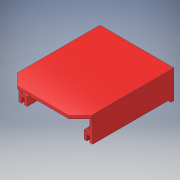
# Autodesk Inventor part: top-slider
Saved by Autodesk Inventor 2018 (Build 220112000, 112)
## iProperties
Created: 2019-10-14
Part Number: top-slider
Material: Generic
Document SubType Name: Modeling
Designer: jklei
Density: 1 g/cm^3
Appearance: Default
Author: jklei
Autodesk Inventor part; units mm, degrees
ref_plane "YZ Plane" through (0, 0, 0) normal (1, 0, 0) x (0, 1, 0)
ref_plane "XZ Plane" through (0, 0, 0) normal (0, 1, 0) x (-1, 0, 0)
ref_plane "XY Plane" through (0, 0, 0) normal (0, 0, 1) x (1, 0, 0)
sketch "Sketch5" plane through (0, 0, 0) normal (0, 0, 1) x (1, 0, 0)
  line L0 (0, 0) -> (82.55, 0)
  line L1 (82.55, 0) -> (82.55, 44.45)
  line L2 (82.55, 44.45) -> (0, 44.45)
  line L3 (0, 44.45) -> (0, 0)
  dimension "d41" = 82.55
  dimension "d42" = 44.45
  constraints: 8 end point, 2 parallel, 1 horizontal, 1 perpendicular
  measures "d41" distance of L2.end L1.end
  measures "d42" distance of L1.end L0.end
extrude "Extrusion5" add sketch "Sketch5" along normal blind 3.175
sketch "Sketch6" plane through (0, 0, 3.175) normal (0, 0, 1) x (1, 0, 0)
  line L0 (0, 0) -> (82.55, 0) projected
  line L1 (82.55, 0) -> (82.55, 44.45) projected
  line L2 (82.55, 44.45) -> (0, 44.45) projected
  line L3 (0, 44.45) -> (0, 0) projected
  line L4 (0, 44.45) -> (0, 0) projected
  line L5 (79.375, 3.175) -> (79.375, 9.525)
  line L6 (79.375, 9.525) -> (76.2, 9.525)
  line L7 (76.2, 9.525) -> (76.2, 3.175)
  line L8 (3.175, 3.175) -> (3.175, 9.525)
  line L9 (3.175, 9.525) -> (6.35, 9.525)
  line L10 (6.35, 9.525) -> (6.35, 3.175)
  line L11 (6.35, 3.175) -> (9.525, 3.175)
  line L12 (9.525, 3.175) -> (9.525, 12.7)
  line L13 (9.525, 12.7) -> (3.175, 12.7)
  line L14 (3.175, 12.7) -> (3.175, 41.275)
  line L15 (3.175, 41.275) -> (79.375, 41.275)
  line L16 (79.375, 41.275) -> (79.375, 12.7)
  line L17 (79.375, 12.7) -> (73.025, 12.7)
  line L18 (73.025, 12.7) -> (73.025, 3.175)
  line L19 (6.35, 3.175) -> (9.525, 3.175)
  line L20 (73.025, 3.175) -> (76.2, 3.175)
  line L21 (0, 44.45) -> (82.55, 44.45)
  line L22 (82.55, 44.45) -> (82.55, 0)
  line L23 (0, 0) -> (0, 44.45)
  line L24 (82.55, 0) -> (82.55, 3.175)
  line L25 (82.55, 0) -> (82.55, 44.45) projected
  line L26 (82.55, 3.175) -> (79.375, 3.175)
  line L27 (0, 0) -> (0, 3.175)
  line L28 (0, 3.175) -> (3.175, 3.175)
  point P0 (3.175, 0)
  dimension "d47" = 6.35
  dimension "d48" = 3.175
  dimension "d51" = 3.175
  dimension "d52" = 3.175
  dimension "d53" = 9.525
  dimension "d54" = 6.35
  dimension "d55" = 28.575
  dimension "d56" = 6.35
  dimension "d61" = 3.175
  dimension "d62" = 3.175
  constraints: 46 end point, 15 perpendicular, 3 point on line, 1 horizontal, 1 parallel, 1 vertical
  measures "d47" distance of L5.start L5.end
  measures "d48" distance of L5.end L6.end
  measures "d51" distance of L8.end L9.end
  measures "d52" distance of L10.end L11.end
  measures "d53" distance of L11.end L12.end
  measures "d54" distance of L12.end L13.end
  measures "d55" distance of L13.end L14.end
  measures "d56" distance of L16.end L17.end
  measures "d61" distance of L0.end L24.end
  measures "d62" distance of L4.end L27.end
extrude "Extrusion7" add sketch "Sketch6" along normal blind 87.5792 contours L3 L2 L1 L26 L5 L6 L7 L20 L18 L17 L16 L15 L14 L13 L12 L11 L10 L9 L8 L28
sketch "Sketch7" plane through (0, 0, 0) normal (0, 0, -1) x (-1, 0, 0)
  line L0 (0, 0) -> (0, 28.575)
  line L1 (0, 44.45) -> (0, 0) projected
  line L2 (0, 28.575) -> (-82.55, 28.575)
  line L3 (-82.55, 0) -> (-82.55, 44.45) projected
  line L4 (-82.55, 28.575) -> (0, 28.575)
  line L5 (0, 28.575) -> (0, 44.45)
  line L6 (0, 44.45) -> (-82.55, 44.45)
  line L7 (-82.55, 44.45) -> (-82.55, 28.575)
  dimension "d63" = 28.575
  constraints: 12 end point, 2 parallel, 2 perpendicular, 2 point on line, 1 horizontal
  measures "d63" distance of L0.start L0.end
extrude "Extrusion8" cut sketch "Sketch7" against normal up to next
sketch "Sketch8" plane through (0, 28.575, 0) normal (0, 1, 0) x (1, 0, 0)
  line L0 (0, 0) -> (82.55, 0) projected
  line L1 (0, 0) -> (82.55, 0)
  line L2 (82.55, -104.775) -> (0, -104.775)
  line L3 (0, -104.775) -> (0, 0)
  line L4 (82.55, 0) -> (82.55, -104.775)
  dimension "d66" = 104.775
  constraints: 8 end point, 1 horizontal, 1 parallel, 1 perpendicular, 1 point on line
  measures "d66" distance of L1.end L2.start
extrude "Extrusion9" add sketch "Sketch8" along normal blind 3.175
chamfer "Chamfer2" distance 12.7 angle 45 2 edges at (82.55, 30.1625, 104.775) (0, 30.1625, 104.775)
body "Solid2"
